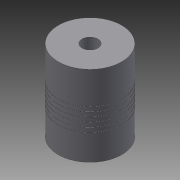
# Autodesk Inventor part: Shaft_Coupler_5mm_10mm
Saved by Autodesk Inventor 2015 (Build 190159000, 159)
## iProperties
Created: 2014-12-22
Part Number: Shaft_Coupler_5mm_10mm
Material: Generic
Document SubType Name: Modeling
Designer: Drew
Density: 1 g/cm^3
Appearance: Default
Author: Drew
Autodesk Inventor part; units mm, degrees
ref_plane "YZ Plane" through (0, 0, 0) normal (1, 0, 0) x (0, 1, 0)
ref_plane "XZ Plane" through (0, 0, 0) normal (0, 1, 0) x (-1, 0, 0)
ref_plane "XY Plane" through (0, 0, 0) normal (0, 0, 1) x (1, 0, 0)
sketch "Sketch2" plane through (0, 0, 0) normal (1, 0, 0) x (0, 1, 0)
  line L0 (3.3337, 0) -> (3.3337, -5)
  line L1 (3.3337, -5) -> (-1.7463, -5)
  line L2 (-1.7463, -5) -> (-1.7463, -10)
  line L3 (23.6537, -10) -> (23.6537, -2.5)
  line L4 (23.6537, -2.5) -> (18.5737, -2.5)
  line L5 (18.5737, -2.5) -> (18.5737, 0)
  line L6 (13.4937, 0) -> (13.4937, -10)
  line L7 (13.3667, -10) -> (13.3667, 0)
  line L8 (18.5737, 0) -> (13.4937, 0)
  line L9 (13.4937, -10) -> (23.6537, -10)
  line L10 (12.0967, 0) -> (12.0967, -10)
  line L11 (11.9697, 0) -> (11.9697, -10)
  line L12 (10.6997, 0) -> (10.6997, -10)
  line L13 (10.5727, 0) -> (10.5727, -10)
  line L14 (12.0967, -10) -> (13.3667, -10)
  line L15 (13.3667, 0) -> (12.0967, 0)
  line L16 (11.9697, 0) -> (10.6997, 0)
  line L17 (10.6997, -10) -> (11.9697, -10)
  line L18 (9.3027, 0) -> (9.3027, -10)
  line L19 (9.1757, -10) -> (9.1757, 0)
  line L20 (7.9057, 0) -> (7.9057, -10)
  line L21 (7.7787, -10) -> (7.7787, 0)
  line L22 (6.5087, 0) -> (6.5087, -10)
  line L23 (6.3817, -10) -> (6.3817, 0)
  line L24 (10.5727, 0) -> (9.3027, 0)
  line L25 (9.3027, -10) -> (10.5727, -10)
  line L26 (7.9057, -10) -> (9.1757, -10)
  line L27 (9.1757, 0) -> (7.9057, 0)
  line L28 (7.7787, 0) -> (6.5087, 0)
  line L29 (6.3817, 0) -> (3.3337, 0)
  line L30 (-1.7463, -10) -> (6.3817, -10)
  line L31 (6.5087, -10) -> (7.7787, -10)
  point P0 (0, 0)
  dimension "d1" = 5.08
  dimension "d2" = 5.08
  dimension "d3" = 25.4
  dimension "d4" = 0.127
  dimension "d5" = 0.127
  dimension "d6" = 0.127
  dimension "d7" = 0.127
  dimension "d8" = 0.127
  dimension "d10" = 0.127
  dimension "d12" = 1.27
  dimension "d13" = 1.27
  dimension "d14" = 1.27
  dimension "d15" = 1.27
  dimension "d16" = 1.27
  dimension "d17" = 2.5
  dimension "d18" = 5
  dimension "d20" = 10
  dimension "d21" = 5.08
  constraints: 86 perpendicular, 64 end point, 7 horizontal, 6 collinear, 2 vertical
  measures "d1" distance of L3.end L4.end
  measures "d2" distance of L0.end L1.end
  measures "d3" distance between parallel lines of L3 L2
  measures "d4" distance between parallel lines of L6 L7
  measures "d5" distance between parallel lines of L11 L10
  measures "d6" distance between parallel lines of L12 L13
  measures "d7" distance between parallel lines of L18 L19
  measures "d8" distance between parallel lines of L20 L21
  measures "d10" distance between parallel lines of L22 L23
  measures "d12" distance between parallel lines of L11 L12
  measures "d13" distance between parallel lines of L13 L18
  measures "d14" distance between parallel lines of L19 L20
  measures "d15" distance between parallel lines of L21 L22
  measures "d16" distance between parallel lines of L7 L10
  measures "d17" distance of L4.end L5.end
  measures "d18" distance of L0.start L0.end
  measures "d20" distance between parallel lines of L8 L9
  measures "d21" distance between parallel lines of L5 L6
revolve "Revolution2" add sketch "Sketch2" angle 360 about axis through (0, 18.5737, 0) along (0, -1, 0)
equation "\"d5\" = d4"
equation "\"d6\" = d5"
equation "\"d7\" = d6"
equation "\"d8\" = d7"
equation "\"d10\" = d8"
equation "\"d13\" = d12"
equation "\"d14\" = d13"
equation "\"d15\" = d14"
equation "\"d16\" = d12"
body "Solid2"
